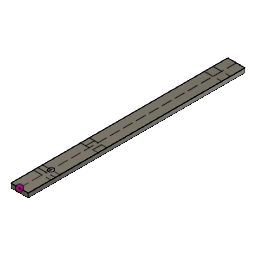
02part (Autodesk Fusion 360 design; units mm, degrees)
Autodesk Fusion 360 part; units mm, degrees
sketch "Sketch4" plane through (0, 0, 0) normal (0, 1, 0) x (1, 0, 0)
  line L0 (-50, 1250) -> (50, 1250)
  line L1 (50, 1250) -> (50, 0)
  line L2 (50, 0) -> (-50, 0)
  line L3 (-50, 0) -> (-50, 1250)
  line L4 (-50, 130) -> (50, 130) construction
  line L5 (-50, 155) -> (50, 155) construction
  line L6 (-50, 182) -> (50, 182) construction
  line L7 (-50, 402) -> (50, 402) construction
  line L8 (-50, 452) -> (50, 452) construction
  line L9 (-50, 1115) -> (50, 1115) construction
  line L10 (-50, 1165) -> (50, 1165) construction
  line L11 (-20, 402) -> (-20, 452) construction
  line L12 (20, 402) -> (20, 452) construction
  line L13 (0, 0) -> (0, 1250) construction
  dimension "d14" = 1250
  dimension "d15" = 100
  dimension "d16" = 130
  dimension "d17" = 25
  dimension "d18" = 27
  dimension "d19" = 220
  dimension "d20" = 50
  dimension "d21" = 40
  dimension "d22" = 960
  dimension "d23" = 50
  constraint horizontal L0
  constraint vertical L1
  constraint horizontal L2
  constraint vertical L3
  constraint coincident L3 L4.start
  constraint coincident L1 L4.end
  constraint perpendicular L1 L4
  constraint coincident L3 L5.start
  constraint coincident L1 L5.end
  constraint perpendicular L1 L5
  constraint coincident L3 L6.start
  constraint coincident L1 L6.end
  constraint perpendicular L1 L6
  constraint coincident L3 L7.start
  constraint coincident L1 L7.end
  constraint perpendicular L1 L7
  constraint coincident L3 L8.start
  constraint coincident L1 L8.end
  constraint perpendicular L1 L8
  constraint coincident L3 L9.start
  constraint coincident L1 L9.end
  constraint perpendicular L1 L9
  constraint coincident L3 L10.start
  constraint coincident L1 L10.end
  constraint perpendicular L1 L10
  constraint coincident L7 L11.start
  constraint coincident L8 L11.end
  constraint perpendicular L8 L11
  constraint coincident L7 L12.start
  constraint coincident L8 L12.end
  constraint perpendicular L8 L12
  constraint midpoint L2 L13.start
  constraint midpoint L0 L13.end
  constraint midpoint L13.start L2
  measures "d14" distance of L0.end L1.end
  measures "d15" distance of L1.end L2.end
  measures "d16" distance of L2 L4
  measures "d17" distance of L4 L5
  measures "d18" distance of L5 L6
  measures "d19" distance of L6 L7
  measures "d20" distance of L7 L8
  measures "d21" distance of L11 L12
  measures "d22" distance of L5 L9
  measures "d23" distance of L9 L10
extrude "Extrude2" add sketch "Sketch4" against normal blind 25
ref_plane "WorkPlane5" through (0, 0, -182) normal (0, -0.92388, 0.382683) x (1, 0, 0)
sketch "Sketch3" plane through (0, 0, -182) normal (0, -0.92388, 0.382683) x (1, 0, 0)
  circle A0 centre (0, 0) radius 15
  dimension "d9" = 30
  constraint coincident A0.centre origin
  measures "d9" diameter of A0
extrude "Extrude3" cut sketch "Sketch3" along normal mid plane 80
equation "d26 = 90 deg - 22.5 deg"
